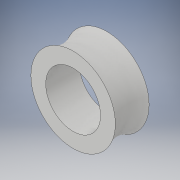
# Autodesk Inventor part: U-Groove-Bearings
Saved by Autodesk Inventor 2017 (Build 210142000, 142)
## iProperties
Created: 2018-10-15
Part Number: U-Groove-Bearings
Material: Generic
Document SubType Name: Modeling
Designer: Tom
Density: 1 g/cm^3
Appearance: Default
Author: Tom
Autodesk Inventor part; units mm, degrees
ref_plane "YZ Plane" through (0, 0, 0) normal (1, 0, 0) x (0, 1, 0)
ref_plane "XZ Plane" through (0, 0, 0) normal (0, 1, 0) x (-1, 0, 0)
ref_plane "XY Plane" through (0, 0, 0) normal (0, 0, 1) x (1, 0, 0)
sketch "Sketch2" plane through (0, 0, 0) normal (0, 1, 0) x (-1, 0, 0)
  arc A0 (7.5, -4) -> (7.5, 4) centre (0, 0) ccw
  line L0 (0, 0) -> (21.3939, 0) construction
  line L1 (7.5, -4) -> (7.5, 4) construction
  line L2 (7.5, -4) -> (17.5, -4)
  line L3 (17.5, -4) -> (17.5, 4)
  line L4 (17.5, 4) -> (7.5, 4)
  point P0 (7.5, 0)
  dimension "d0" = 17
  dimension "d1" = 8
  dimension "d3" = 10
  dimension "d4" = 8
  dimension "d5" = 17.5
  constraints: 10 end point, 2 point on circle, 1 centre point, 1 coincident, 1 horizontal, 1 midpoint, 1 perpendicular, 1 point on line, 1 vertical
  measures "d0" diameter of A0
  measures "d1" distance of L1.start L1.end
  measures "d3" distance of L1.start L2.end
  measures "d4" distance of L2.end L3.end
  measures "d5" distance from line of point (0, 0) L3
revolve "Revolution1" add sketch "Sketch2" angle 360 about axis through (-17.5, 0, -4) along (0, 0, 1)
hole "Hole1" at (-17.5, 0, 4) direction (0, 0, -1) diameter 13 end through all
body "Solid1"
